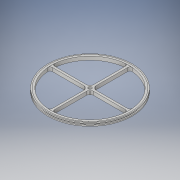
# Autodesk Inventor part: MTV Front Brake Axle (11.19)
Saved by Autodesk Inventor 2018 (Build 220112000, 112)
## iProperties
Created: 2018-11-20
Part Number: MTV Front Brake Axle (11.19)
Material: Generic
Document SubType Name: Modeling
Designer: Aditya Kendre
Density: 1 g/cm^3
Appearance: Default
Author: Aditya Kendre
## iProperties of the stored document MTV Front Brake Axle (11_3DPrint.ipt
Created: 2018-11-27
Part Number: MTV Front Brake Axle (11_3DPrint
Material: Generic
Document SubType Name: Modeling
Designer: Aditya Kendre
Density: 1 g/cm^3
Appearance: Default
Author: Aditya Kendre
Autodesk Inventor part; units mm, degrees
ref_plane "YZ Plane" through (0, 0, 0) normal (1, 0, 0) x (0, 1, 0)
ref_plane "XZ Plane" through (0, 0, 0) normal (0, 1, 0) x (-1, 0, 0)
ref_plane "XY Plane" through (0, 0, 0) normal (0, 0, 1) x (1, 0, 0)
sketch "Sketch1" plane through (0, 0, 0) normal (0, 1, 0) x (-1, 0, 0)
  circle A0 centre (0, 0) radius 60
  circle A1 centre (0, 0) radius 61.5823
  dimension "d0" = 120
  dimension "d1" = 123.1646
  constraints: 2 centre point, 2 coincident
  measures "d0" diameter of A0
  measures "d1" diameter of A1
extrude "Extrusion1" add sketch "Sketch1" along normal blind 1.5875
sketch "Sketch2" plane through (0, 1.5875, 0) normal (0, 1, 0) x (1, 0, 0)
  circle A0 centre (0, 0) radius 60
  circle A1 centre (0, 0) radius 57.15
  dimension "d4" = 114.3
  constraints: 2 centre point, 2 coincident
  measures "d4" diameter of A1
extrude "Extrusion2" add sketch "Sketch2" along normal blind 2
sketch "Sketch3" plane through (0, 3.5875, 0) normal (0, 1, 0) x (1, 0, 0)
  circle A0 centre (0, 0) radius 60
  circle A1 centre (0, 0) radius 61.5823
  constraints: 2 centre point, 2 coincident
extrude "Extrusion3" add sketch "Sketch3" along normal blind 1.5875
sketch "Sketch4" plane through (0, 0, 0) normal (0, -1, 0) x (1, 0, 0)
  circle A0 centre (0, 0) radius 60
  constraints: 1 centre point, 1 coincident
extrude "Extrusion4" add sketch "Sketch4" against normal blind 5.1816
sketch "Sketch5" plane through (0, 5.1816, 0) normal (0, 1, 0) x (1, 0, 0)
  circle A0 centre (0, 0) radius 57.15
  dimension "d11" = 114.3
  constraints: 1 centre point, 1 coincident
  measures "d11" diameter of A0
extrude "Extrusion5" cut sketch "Sketch5" against normal blind 5.1816
sketch "Sketch6" plane through (0, 5.175, 0) normal (0, 1, 0) x (1, 0, 0)
  circle A0 centre (0, 0) radius 2.4765
  circle A1 centre (0, 0) radius 5.1008
  dimension "d14" = 4.953
  constraints: 2 centre point, 2 coincident
  measures "d14" diameter of A0
extrude "Extrusion6" add sketch "Sketch6" against normal blind 5.1816
sketch "Sketch7" plane through (0, -0.0066, 0) normal (0, -1, 0) x (1, 0, 0)
  circle A0 centre (0, 0) radius 5.1008 projected
  circle A1 centre (0, 0) radius 57.15 projected
  line L0 (-3.0273, 1.5838) -> (-58.1435, 1.5838)
  line L1 (-58.1435, 1.5838) -> (-58.1435, -1.5838)
  line L2 (-58.1435, -1.5838) -> (-3.0273, -1.5838)
  line L3 (-3.0273, -1.5838) -> (-3.0273, 1.5838)
  line L4 (-3.0273, 1.5838) -> (-58.1435, -1.5838) construction
  line L5 (-58.1435, 1.5838) -> (-3.0273, -1.5838) construction
  line L6 (1.5875, 58.4929) -> (-1.5875, 58.4929)
  line L7 (-1.5875, 58.4929) -> (-1.5875, 3.6522)
  line L8 (-1.5875, 3.6522) -> (1.5875, 3.6522)
  line L9 (1.5875, 3.6522) -> (1.5875, 58.4929)
  line L10 (1.5875, 58.4929) -> (-1.5875, 3.6522) construction
  line L11 (-1.5875, 58.4929) -> (1.5875, 3.6522) construction
  line L12 (58.6337, -1.5875) -> (3.4947, -1.5875)
  line L13 (3.4947, -1.5875) -> (3.4947, 1.5875)
  line L14 (3.4947, 1.5875) -> (58.6337, 1.5875)
  line L15 (58.6337, 1.5875) -> (58.6337, -1.5875)
  line L16 (58.6337, -1.5875) -> (3.4947, 1.5875) construction
  line L17 (3.4947, -1.5875) -> (58.6337, 1.5875) construction
  line L18 (1.5875, -3.7293) -> (-1.5875, -3.7293)
  line L19 (-1.5875, -3.7293) -> (-1.5875, -58.3991)
  line L20 (-1.5875, -58.3991) -> (1.5875, -58.3991)
  line L21 (1.5875, -58.3991) -> (1.5875, -3.7293)
  line L22 (1.5875, -3.7293) -> (-1.5875, -58.3991) construction
  line L23 (-1.5875, -3.7293) -> (1.5875, -58.3991) construction
  point P0 (-30.5854, 0)
  point P1 (0, 31.0726)
  point P2 (31.0642, 0)
  point P3 (0, -31.0642)
  dimension "d17" = 3.175
  dimension "d18" = 3.175
  constraints: 48 end point, 8 midpoint, 8 parallel, 4 horizontal, 4 perpendicular, 1 point on line
  measures "d17" distance of L8.end L7.end
  measures "d18" distance of L12.end L13.end
extrude "Extrusion7" add sketch "Sketch7" against normal blind 5.1816 contours A0 L12 L13 L14 | A0 L14 A1 L12 | L9 L8 L7 A0 | A0 L7 A1 L9 | L14 L15 L12 A1 | L21 A1 L19 A0 | A0 L19 L18 L21 | A1 L7 L6 L9 | L21 L20 L19 A1 | L0 L3 L2 A0 | A0 L2 A1 L0 | A1 L2 L1 L0
fillet "Fillet1" radius 3.175 8 edges at (57.1279, 2.5875, 1.5875) (57.1279, 2.5875, -1.5875) (-1.5875, 2.5875, 57.1279) (1.5875, 2.5875, 57.1279) (-57.128, 2.5875, 1.5838) (-57.128, 2.5875, -1.5838) (-1.5875, 2.5875, -57.1279) (1.5875, 2.5875, -57.1279)
fillet "Fillet2" radius 3.175 8 edges at (4.8475, 2.5842, -1.5875) (1.5875, 2.5842, -4.8475) (-1.5875, 2.5842, 4.8475) (-4.8487, 2.5842, 1.5838) (-1.5875, 2.5842, -4.8475) (-4.8487, 2.5842, -1.5838) (4.8475, 2.5842, 1.5875) (1.5875, 2.5842, 4.8475)
body "Solid1"
